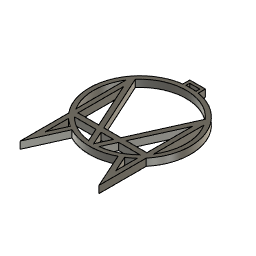
Homework 1.a v1 (Autodesk Fusion 360 design; units mm, degrees)
Autodesk Fusion 360 part; units mm, degrees
note: some values were not read from the file. Set by a fixed rule: which sketch regions a step uses.
sketch "Sketch1" plane through (0, 0, 0) normal (0, 0, 1) x (1, 0, 0)
  circle A0 centre (0, 11) radius 32.5228
  circle A1 centre (0, 11) radius 35.5057
  line L0 (27.2057, -11.8146) -> (27.2057, -45)
  line L1 (27.2057, -45) -> (16.1805, -20.6046)
  line L2 (24.1506, -15.027) -> (24.1506, -30)
  line L3 (24.1506, -30) -> (19.1372, -18.9069)
  line L4 (-16.1421, -20.6242) -> (-27.4351, -45.7523)
  line L5 (-27.4351, -45.7523) -> (-27.4351, 28.4657)
  line L6 (27.4351, 28.4657) -> (27.2057, -45)
  line L7 (24.15, 23.7181) -> (24.1506, -30)
  line L8 (24.15, 23.7181) -> (3.6905, -21.3128)
  line L9 (-3.6905, -21.3128) -> (-24.2501, 23.7181)
  line L10 (-24.2501, 23.7181) -> (-24.2495, -31.0996)
  line L11 (-24.2495, -31.0996) -> (-18.8513, -19.088)
  line L12 (0, -21.5228) -> (24.3204, 32.5929)
  line L13 (0, -21.5228) -> (-24.5749, 32.3028)
  line L14 (23.0617, -11.9324) -> (-23.0612, -11.9329)
  line L15 (26.1993, -8.27) -> (-24.2497, -8.2706)
  line L16 (-5, 44) -> (6, 44)
  line L17 (6, 44) -> (6, 51)
  line L18 (6, 51) -> (-5, 51)
  line L19 (-5, 51) -> (-5, 44)
  line L20 (4, 49) -> (-3, 49)
  line L21 (-3, 49) -> (-3, 46.3788)
  line L22 (-3, 46.3788) -> (4, 46.3788)
  line L23 (4, 46.3788) -> (4, 49)
  dimension "d3" = 7
  constraint concentric A0 A1
  constraint coincident A1 L0.start
  constraint vertical L0
  constraint coincident A1 L1.end
  constraint coincident A1 L2.start
  constraint parallel L0 L2
  constraint coincident A1 L3.end
  constraint parallel L1 L3
  constraint coincident A1 L4.start
  constraint coincident A0 L5.end
  constraint vertical L5
  constraint coincident A0 L6.start
  constraint coincident A0 L8.end
  constraint coincident A0 L9.start
  constraint parallel L7 L10
  constraint coincident A1 L11.end
  constraint parallel L4 L11
  constraint coincident A0 L12.start
  constraint coincident A0 L12.end
  constraint parallel L11 L12
  constraint coincident A0 L13.end
  constraint parallel L9 L13
  constraint coincident A0 L14.start
  constraint coincident A0 L14.end
  constraint perpendicular L10 L14
  constraint coincident L10 L15.end
  constraint perpendicular L10 L15
  constraint horizontal L16
  constraint vertical L17
  constraint horizontal L18
  constraint vertical L19
  constraint horizontal L20
  constraint vertical L21
  constraint horizontal L22
  constraint vertical L23
  constraint coincident A1 L21.end
  measures "d3" distance of L20.start L20.end
extrude "Extrude1" add sketch "Sketch1" along normal blind 5 contours A0 A1 L5 L6 L16 L17 L19 | A0 L6 L7 L8 L12 L15 | A0 A1 L6 L7 | A0 L7 L15 | A0 L5 L9 L10 L13 L15 | L8 L12 L14 L15 | L12 L13 L14 L15 | A0 A1 L7 L10 | A0 L7 L8 L14 L15 | A1 L0 L1 L2 L3 L7 | L9 L13 L14 L15 | A0 L8 L12 L14 | A1 L16 L17 L19 L22 | A0 A1 L5 L10 | A0 L9 L13 L14 | A0 L9 L10 L14 L15 | A1 L22 | A1 L4 L5 L10 L11
extrude "Extrude2" add sketch "Sketch1" along normal blind 5 contours A1 L16 L17 L19 L22 | A1 L17 L18 L19 L20 L21 L22 L23
